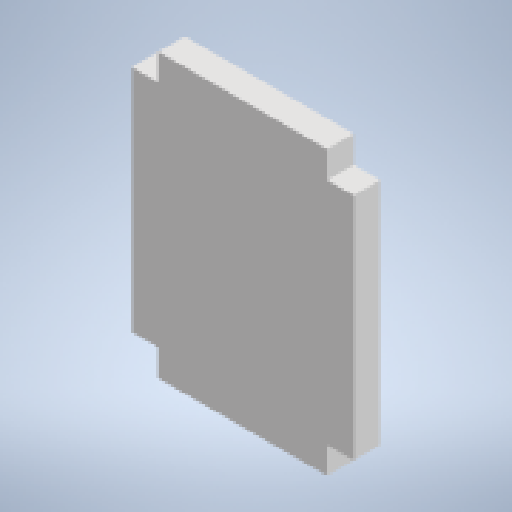
# Autodesk Inventor part: servo short side
Saved by Autodesk Inventor 2023 (Build 270158000, 158)
## iProperties
Created: 2023-11-14
Part Number: servo short side
Material: Generic
Document SubType Name: Modeling
Designer: Nate
Density: 1 g/cm^3
Appearance: Default
Author: Nate
Autodesk Inventor part; units mm, degrees
ref_plane "YZ Plane" through (0, 0, 0) normal (1, 0, 0) x (0, 1, 0)
ref_plane "XZ Plane" through (0, 0, 0) normal (0, 1, 0) x (-1, 0, 0)
ref_plane "XY Plane" through (0, 0, 0) normal (0, 0, 1) x (1, 0, 0)
sketch "Sketch1" plane through (0, 0, 0) normal (0, 0, 1) x (1, 0, 0)
  line L0 (0, 0) -> (-20.066, 0)
  line L1 (-20.066, 0) -> (-20.066, -33.6042)
  line L2 (-20.066, -33.6042) -> (0, -33.6042)
  line L3 (0, -33.6042) -> (0, 0)
  line L4 (0, -3.175) -> (3.175, -3.175)
  line L5 (3.175, -3.175) -> (3.175, -30.4292)
  line L6 (3.175, -30.4292) -> (0, -30.4292)
  line L7 (0, -30.4292) -> (0, -3.175)
  line L8 (-20.066, -3.175) -> (-23.241, -3.175)
  line L9 (-23.241, -3.175) -> (-23.241, -30.4292)
  line L10 (-23.241, -30.4292) -> (-20.066, -30.4292)
  line L11 (-20.066, -30.4292) -> (-20.066, -3.175)
  point P0 (1.5875, -30.4292)
  point P1 (0, -30.4292)
  dimension "d0" = 3.175
  dimension "d1" = 3.175
  dimension "d2" = 3.175
  dimension "d3" = 3.175
  dimension "d4" = 3.175
  dimension "d6" = 3.175
  dimension "d7" = 27.2542
  dimension "d8" = 20.066
  constraints: 24 end point, 6 parallel, 3 horizontal, 3 perpendicular, 2 point on line, 1 midpoint
  measures "d0" distance between parallel lines of L4 L0
  measures "d1" distance between parallel lines of L3 L5
  measures "d2" distance between parallel lines of L1 L9
  measures "d3" distance between parallel lines of L0 L8
  measures "d4" distance between parallel lines of L2 L10
  measures "d6" distance from line of L2 point (1.588, -30.429)
  measures "d7" distance between parallel lines of L6 L4
  measures "d8" distance between parallel lines of L3 L1
extrude "Extrusion1" add sketch "Sketch1" along normal blind 3.175
body "Solid1"
